Autodesk Inventor part; units mm, degrees
(part 2 of 2)
sketch "Sketch6" plane through (-19, 24.5, 7) normal (0, 0, 1) x (1, 0, 0)
  line L0 (58.5, 3.5) -> (-18, 3.5) projected
  line L1 (-18, 11.1) -> (-18, 3.5) projected
  line L2 (-24, 11.1) -> (-18, 11.1) projected
  line L3 (-24, 11.1) -> (-24, -60.3239) projected
  line L4 (-24, -60.3239) -> (-18, -60.3239) projected
  line L5 (-18, -52.5) -> (-18, -60.3239) projected
  line L6 (-18, -52.5) -> (58.5, -52.5) projected
  arc A0 (58.5, -52.5) -> (61.5, -49.5) centre (58.5, -49.5) ccw projected
  line L7 (61.5, -49.5) -> (61.5, 0.5) projected
  arc A1 (61.5, 0.5) -> (58.5, 3.5) centre (58.5, 0.5) ccw projected
  line L8 (-13.9349, -14.3893) -> (-16.5478, -12.8807) projected
  line L9 (-16.5478, -12.8807) -> (-16.5478, -9.8635) projected
  line L10 (-16.5478, -9.8635) -> (-13.9349, -8.3549) projected
  line L11 (-13.9349, -8.3549) -> (-11.3219, -9.8635) projected
  line L12 (-11.3219, -9.8635) -> (-11.3219, -12.8807) projected
  line L13 (-11.3219, -12.8807) -> (-13.9349, -14.3893) projected
  line L14 (-16.5478, -17.8635) -> (-13.9349, -16.3549) projected
  line L15 (-13.9349, -16.3549) -> (-11.3219, -17.8635) projected
  line L16 (-11.3219, -17.8635) -> (-11.3219, -20.8807) projected
  line L17 (-11.3219, -20.8807) -> (-13.9349, -22.3893) projected
  line L18 (-13.9349, -22.3893) -> (-16.5478, -20.8807) projected
  line L19 (-16.5478, -20.8807) -> (-16.5478, -17.8635) projected
  line L20 (-16.5478, -25.8635) -> (-13.9349, -24.3549) projected
  line L21 (-13.9349, -24.3549) -> (-11.3219, -25.8635) projected
  line L22 (-11.3219, -25.8635) -> (-11.3219, -28.8807) projected
  line L23 (-11.3219, -28.8807) -> (-13.9349, -30.3893) projected
  line L24 (-13.9349, -30.3893) -> (-16.5478, -28.8807) projected
  line L25 (-16.5478, -28.8807) -> (-16.5478, -25.8635) projected
  line L26 (-16.5478, -33.8635) -> (-13.9349, -32.3549) projected
  line L27 (-13.9349, -32.3549) -> (-11.3219, -33.8635) projected
  line L28 (-11.3219, -33.8635) -> (-11.3219, -36.8807) projected
  line L29 (-11.3219, -36.8807) -> (-13.9349, -38.3893) projected
  line L30 (-13.9349, -38.3893) -> (-16.5478, -36.8807) projected
  line L31 (-16.5478, -36.8807) -> (-16.5478, -33.8635) projected
  line L32 (-16.5478, -41.8635) -> (-13.9349, -40.3549) projected
  line L33 (-13.9349, -40.3549) -> (-11.3219, -41.8635) projected
  line L34 (-11.3219, -41.8635) -> (-11.3219, -44.8807) projected
  line L35 (-11.3219, -44.8807) -> (-13.9349, -46.3893) projected
  line L36 (-13.9349, -46.3893) -> (-15.4751, -45.5) projected
  line L37 (-15.4751, -45.5) -> (-16.5, -45.5) projected
  line L38 (-16.5, -45.5) -> (-16.5, -44.9083) projected
  line L39 (-16.5, -44.9083) -> (-16.5478, -44.8807) projected
  line L40 (-16.5478, -44.8807) -> (-16.5478, -41.8635) projected
  line L41 (-8.8465, -45.5) -> (-6.8631, -44.3549) projected
  line L42 (-6.8631, -44.3549) -> (-4.8796, -45.5) projected
  line L43 (-4.8796, -45.5) -> (-8.8465, -45.5) projected
  line L44 (0.0651, -46.3893) -> (-2.5478, -44.8807) projected
  line L45 (-2.5478, -44.8807) -> (-2.5478, -41.8635) projected
  line L46 (-2.5478, -41.8635) -> (0.0651, -40.3549) projected
  line L47 (0.0651, -40.3549) -> (2.6781, -41.8635) projected
  line L48 (2.6781, -41.8635) -> (2.6781, -44.8807) projected
  line L49 (2.6781, -44.8807) -> (0.0651, -46.3893) projected
  line L50 (5.1535, -45.5) -> (7.1369, -44.3549) projected
  line L51 (7.1369, -44.3549) -> (9.1204, -45.5) projected
  line L52 (9.1204, -45.5) -> (5.1535, -45.5) projected
  line L53 (14.0651, -46.3893) -> (11.4522, -44.8807) projected
  line L54 (11.4522, -44.8807) -> (11.4522, -41.8635) projected
  line L55 (11.4522, -41.8635) -> (14.0651, -40.3549) projected
  line L56 (14.0651, -40.3549) -> (16.6781, -41.8635) projected
  line L57 (16.6781, -41.8635) -> (16.6781, -44.8807) projected
  line L58 (16.6781, -44.8807) -> (14.0651, -46.3893) projected
  line L59 (19.1535, -45.5) -> (21.1369, -44.3549) projected
  line L60 (21.1369, -44.3549) -> (23.1204, -45.5) projected
  line L61 (23.1204, -45.5) -> (19.1535, -45.5) projected
  line L62 (28.0651, -46.3893) -> (25.4522, -44.8807) projected
  line L63 (25.4522, -44.8807) -> (25.4522, -41.8635) projected
  line L64 (25.4522, -41.8635) -> (28.0651, -40.3549) projected
  line L65 (28.0651, -40.3549) -> (30.6781, -41.8635) projected
  line L66 (30.6781, -41.8635) -> (30.6781, -44.8807) projected
  line L67 (30.6781, -44.8807) -> (28.0651, -46.3893) projected
  line L68 (33.1535, -45.5) -> (35.1369, -44.3549) projected
  line L69 (35.1369, -44.3549) -> (37.1204, -45.5) projected
  line L70 (37.1204, -45.5) -> (33.1535, -45.5) projected
  line L71 (42.0651, -46.3893) -> (39.4522, -44.8807) projected
  line L72 (39.4522, -44.8807) -> (39.4522, -41.8635) projected
  line L73 (39.4522, -41.8635) -> (42.0651, -40.3549) projected
  line L74 (42.0651, -40.3549) -> (44.6781, -41.8635) projected
  line L75 (44.6781, -41.8635) -> (44.6781, -44.8807) projected
  line L76 (44.6781, -44.8807) -> (42.0651, -46.3893) projected
  line L77 (47.1535, -45.5) -> (49.1369, -44.3549) projected
  line L78 (49.1369, -44.3549) -> (51.1204, -45.5) projected
  line L79 (51.1204, -45.5) -> (47.1535, -45.5) projected
  line L80 (54.5, -45.4856) -> (53.4522, -44.8807) projected
  line L81 (53.4522, -44.8807) -> (53.4522, -41.8635) projected
  line L82 (53.4522, -41.8635) -> (54.5, -41.2585) projected
  line L83 (54.5, -41.2585) -> (54.5, -45.4856) projected
  line L84 (54.5, -37.4856) -> (53.4522, -36.8807) projected
  line L85 (53.4522, -36.8807) -> (53.4522, -33.8635) projected
  line L86 (53.4522, -33.8635) -> (54.5, -33.2585) projected
  line L87 (54.5, -33.2585) -> (54.5, -37.4856) projected
  line L88 (54.5, -29.4856) -> (53.4522, -28.8807) projected
  line L89 (53.4522, -28.8807) -> (53.4522, -25.8635) projected
  line L90 (53.4522, -25.8635) -> (54.5, -25.2585) projected
  line L91 (54.5, -25.2585) -> (54.5, -29.4856) projected
  line L92 (54.5, -21.4856) -> (53.4522, -20.8807) projected
  line L93 (53.4522, -20.8807) -> (53.4522, -17.8635) projected
  line L94 (53.4522, -17.8635) -> (54.5, -17.2585) projected
  line L95 (54.5, -17.2585) -> (54.5, -21.4856) projected
  line L96 (54.5, -13.4856) -> (53.4522, -12.8807) projected
  line L97 (53.4522, -12.8807) -> (53.4522, -9.8635) projected
  line L98 (53.4522, -9.8635) -> (54.5, -9.2585) projected
  line L99 (54.5, -9.2585) -> (54.5, -13.4856) projected
  line L100 (54.5, -5.4856) -> (53.4522, -4.8807) projected
  line L101 (53.4522, -4.8807) -> (53.4522, -3.5) projected
  line L102 (53.4522, -3.5) -> (54.5, -3.5) projected
  line L103 (54.5, -3.5) -> (54.5, -5.4856) projected
  line L104 (44.6781, -3.5) -> (44.6781, -4.8807) projected
  line L105 (44.6781, -4.8807) -> (42.0651, -6.3893) projected
  line L106 (42.0651, -6.3893) -> (39.4522, -4.8807) projected
  line L107 (39.4522, -4.8807) -> (39.4522, -3.5) projected
  line L108 (39.4522, -3.5) -> (44.6781, -3.5) projected
  line L109 (30.6781, -3.5) -> (30.6781, -4.8807) projected
  line L110 (30.6781, -4.8807) -> (28.0651, -6.3893) projected
  line L111 (28.0651, -6.3893) -> (25.4522, -4.8807) projected
  line L112 (25.4522, -4.8807) -> (25.4522, -3.5) projected
  line L113 (25.4522, -3.5) -> (30.6781, -3.5) projected
  line L114 (16.6781, -3.5) -> (16.6781, -4.8807) projected
  line L115 (16.6781, -4.8807) -> (14.0651, -6.3893) projected
  line L116 (14.0651, -6.3893) -> (11.4522, -4.8807) projected
  line L117 (11.4522, -4.8807) -> (11.4522, -3.5) projected
  line L118 (11.4522, -3.5) -> (16.6781, -3.5) projected
  line L119 (2.6781, -3.5) -> (2.6781, -4.8807) projected
  line L120 (2.6781, -4.8807) -> (0.0651, -6.3893) projected
  line L121 (0.0651, -6.3893) -> (-2.5478, -4.8807) projected
  line L122 (-2.5478, -4.8807) -> (-2.5478, -3.5) projected
  line L123 (-2.5478, -3.5) -> (2.6781, -3.5) projected
  line L124 (7.1369, -10.3893) -> (4.524, -8.8807) projected
  line L125 (4.524, -8.8807) -> (4.524, -5.8635) projected
  line L126 (4.524, -5.8635) -> (7.1369, -4.3549) projected
  line L127 (7.1369, -4.3549) -> (9.7499, -5.8635) projected
  line L128 (9.7499, -5.8635) -> (9.7499, -8.8807) projected
  line L129 (9.7499, -8.8807) -> (7.1369, -10.3893) projected
  line L130 (7.1369, -18.3893) -> (4.524, -16.8807) projected
  line L131 (4.524, -16.8807) -> (4.524, -13.8635) projected
  line L132 (4.524, -13.8635) -> (7.1369, -12.3549) projected
  line L133 (7.1369, -12.3549) -> (9.7499, -13.8635) projected
  line L134 (9.7499, -13.8635) -> (9.7499, -16.8807) projected
  line L135 (9.7499, -16.8807) -> (7.1369, -18.3893) projected
  line L136 (-6.8631, -18.3893) -> (-9.476, -16.8807) projected
  line L137 (-9.476, -16.8807) -> (-9.476, -13.8635) projected
  line L138 (-9.476, -13.8635) -> (-6.8631, -12.3549) projected
  line L139 (-6.8631, -12.3549) -> (-4.2501, -13.8635) projected
  line L140 (-4.2501, -13.8635) -> (-4.2501, -16.8807) projected
  line L141 (-4.2501, -16.8807) -> (-6.8631, -18.3893) projected
  line L142 (-6.8631, -10.3893) -> (-9.476, -8.8807) projected
  line L143 (-9.476, -8.8807) -> (-9.476, -5.8635) projected
  line L144 (-9.476, -5.8635) -> (-6.8631, -4.3549) projected
  line L145 (-6.8631, -4.3549) -> (-4.2501, -5.8635) projected
  line L146 (-4.2501, -5.8635) -> (-4.2501, -8.8807) projected
  line L147 (-4.2501, -8.8807) -> (-6.8631, -10.3893) projected
  line L148 (9.7499, -24.8807) -> (7.1369, -26.3893) projected
  line L149 (7.1369, -26.3893) -> (4.524, -24.8807) projected
  line L150 (4.524, -24.8807) -> (4.524, -21.8635) projected
  line L151 (4.524, -21.8635) -> (7.1369, -20.3549) projected
  line L152 (7.1369, -20.3549) -> (9.7499, -21.8635) projected
  line L153 (9.7499, -21.8635) -> (9.7499, -24.8807) projected
  line L154 (9.7499, -32.8807) -> (7.1369, -34.3893) projected
  line L155 (7.1369, -34.3893) -> (4.524, -32.8807) projected
  line L156 (4.524, -32.8807) -> (4.524, -29.8635) projected
  line L157 (4.524, -29.8635) -> (7.1369, -28.3549) projected
  line L158 (7.1369, -28.3549) -> (9.7499, -29.8635) projected
  line L159 (9.7499, -29.8635) -> (9.7499, -32.8807) projected
  line L160 (9.7499, -40.8807) -> (7.1369, -42.3893) projected
  line L161 (7.1369, -42.3893) -> (4.524, -40.8807) projected
  line L162 (4.524, -40.8807) -> (4.524, -37.8635) projected
  line L163 (4.524, -37.8635) -> (7.1369, -36.3549) projected
  line L164 (7.1369, -36.3549) -> (9.7499, -37.8635) projected
  line L165 (9.7499, -37.8635) -> (9.7499, -40.8807) projected
  line L166 (16.6781, -12.8807) -> (14.0651, -14.3893) projected
  line L167 (14.0651, -14.3893) -> (11.4522, -12.8807) projected
  line L168 (11.4522, -12.8807) -> (11.4522, -9.8635) projected
  line L169 (11.4522, -9.8635) -> (14.0651, -8.3549) projected
  line L170 (14.0651, -8.3549) -> (16.6781, -9.8635) projected
  line L171 (16.6781, -9.8635) -> (16.6781, -12.8807) projected
  line L172 (16.6781, -20.8807) -> (14.0651, -22.3893) projected
  line L173 (14.0651, -22.3893) -> (11.4522, -20.8807) projected
  line L174 (11.4522, -20.8807) -> (11.4522, -17.8635) projected
  line L175 (11.4522, -17.8635) -> (14.0651, -16.3549) projected
  line L176 (14.0651, -16.3549) -> (16.6781, -17.8635) projected
  line L177 (16.6781, -17.8635) -> (16.6781, -20.8807) projected
  line L178 (16.6781, -28.8807) -> (14.0651, -30.3893) projected
  line L179 (14.0651, -30.3893) -> (11.4522, -28.8807) projected
  line L180 (11.4522, -28.8807) -> (11.4522, -25.8635) projected
  line L181 (11.4522, -25.8635) -> (14.0651, -24.3549) projected
  line L182 (14.0651, -24.3549) -> (16.6781, -25.8635) projected
  line L183 (16.6781, -25.8635) -> (16.6781, -28.8807) projected
  line L184 (16.6781, -36.8807) -> (14.0651, -38.3893) projected
  line L185 (14.0651, -38.3893) -> (11.4522, -36.8807) projected
  line L186 (11.4522, -36.8807) -> (11.4522, -33.8635) projected
  line L187 (11.4522, -33.8635) -> (14.0651, -32.3549) projected
  line L188 (14.0651, -32.3549) -> (16.6781, -33.8635) projected
  line L189 (16.6781, -33.8635) -> (16.6781, -36.8807) projected
  line L190 (23.7499, -5.8635) -> (23.7499, -8.8807) projected
  line L191 (23.7499, -8.8807) -> (21.1369, -10.3893) projected
  line L192 (21.1369, -10.3893) -> (18.524, -8.8807) projected
  line L193 (18.524, -8.8807) -> (18.524, -5.8635) projected
  line L194 (18.524, -5.8635) -> (21.1369, -4.3549) projected
  line L195 (21.1369, -4.3549) -> (23.7499, -5.8635) projected
  line L196 (18.524, -40.8807) -> (18.524, -37.8635) projected
  line L197 (18.524, -37.8635) -> (21.1369, -36.3549) projected
  line L198 (21.1369, -36.3549) -> (23.7499, -37.8635) projected
  line L199 (23.7499, -37.8635) -> (23.7499, -40.8807) projected
  line L200 (23.7499, -40.8807) -> (21.1369, -42.3893) projected
  line L201 (21.1369, -42.3893) -> (18.524, -40.8807) projected
  line L202 (25.4522, -20.8807) -> (25.4522, -17.8635) projected
  line L203 (25.4522, -17.8635) -> (28.0651, -16.3549) projected
  line L204 (28.0651, -16.3549) -> (30.6781, -17.8635) projected
  line L205 (30.6781, -17.8635) -> (30.6781, -20.8807) projected
  line L206 (30.6781, -20.8807) -> (28.0651, -22.3893) projected
  line L207 (28.0651, -22.3893) -> (25.4522, -20.8807) projected
  line L208 (28.0651, -14.3893) -> (25.4522, -12.8807) projected
  line L209 (25.4522, -12.8807) -> (25.4522, -9.8635) projected
  line L210 (25.4522, -9.8635) -> (28.0651, -8.3549) projected
  line L211 (28.0651, -8.3549) -> (30.6781, -9.8635) projected
  line L212 (30.6781, -9.8635) -> (30.6781, -12.8807) projected
  line L213 (30.6781, -12.8807) -> (28.0651, -14.3893) projected
  line L214 (25.4522, -25.8635) -> (28.0651, -24.3549) projected
  line L215 (28.0651, -24.3549) -> (30.6781, -25.8635) projected
  line L216 (30.6781, -25.8635) -> (30.6781, -28.8807) projected
  line L217 (30.6781, -28.8807) -> (28.0651, -30.3893) projected
  line L218 (28.0651, -30.3893) -> (25.4522, -28.8807) projected
  line L219 (25.4522, -28.8807) -> (25.4522, -25.8635) projected
  line L220 (28.0651, -32.3549) -> (30.6781, -33.8635) projected
  line L221 (30.6781, -33.8635) -> (30.6781, -36.8807) projected
  line L222 (30.6781, -36.8807) -> (28.0651, -38.3893) projected
  line L223 (28.0651, -38.3893) -> (25.4522, -36.8807) projected
  line L224 (25.4522, -36.8807) -> (25.4522, -33.8635) projected
  line L225 (25.4522, -33.8635) -> (28.0651, -32.3549) projected
  line L226 (23.7499, -24.8807) -> (21.1369, -26.3893) projected
  line L227 (21.1369, -26.3893) -> (18.524, -24.8807) projected
  line L228 (18.524, -24.8807) -> (18.524, -21.8635) projected
  line L229 (18.524, -21.8635) -> (21.1369, -20.3549) projected
  line L230 (21.1369, -20.3549) -> (23.7499, -21.8635) projected
  line L231 (23.7499, -21.8635) -> (23.7499, -24.8807) projected
  line L232 (23.7499, -32.8807) -> (21.1369, -34.3893) projected
  line L233 (21.1369, -34.3893) -> (18.524, -32.8807) projected
  line L234 (18.524, -32.8807) -> (18.524, -29.8635) projected
  line L235 (18.524, -29.8635) -> (21.1369, -28.3549) projected
  line L236 (21.1369, -28.3549) -> (23.7499, -29.8635) projected
  line L237 (23.7499, -29.8635) -> (23.7499, -32.8807) projected
  line L238 (23.7499, -16.8807) -> (21.1369, -18.3893) projected
  line L239 (21.1369, -18.3893) -> (18.524, -16.8807) projected
  line L240 (18.524, -16.8807) -> (18.524, -13.8635) projected
  line L241 (18.524, -13.8635) -> (21.1369, -12.3549) projected
  line L242 (21.1369, -12.3549) -> (23.7499, -13.8635) projected
  line L243 (23.7499, -13.8635) -> (23.7499, -16.8807) projected
  line L244 (37.7499, -5.8635) -> (37.7499, -8.8807) projected
  line L245 (37.7499, -8.8807) -> (35.1369, -10.3893) projected
  line L246 (35.1369, -10.3893) -> (32.524, -8.8807) projected
  line L247 (32.524, -8.8807) -> (32.524, -5.8635) projected
  line L248 (32.524, -5.8635) -> (35.1369, -4.3549) projected
  line L249 (35.1369, -4.3549) -> (37.7499, -5.8635) projected
  line L250 (32.524, -40.8807) -> (32.524, -37.8635) projected
  line L251 (32.524, -37.8635) -> (35.1369, -36.3549) projected
  line L252 (35.1369, -36.3549) -> (37.7499, -37.8635) projected
  line L253 (37.7499, -37.8635) -> (37.7499, -40.8807) projected
  line L254 (37.7499, -40.8807) -> (35.1369, -42.3893) projected
  line L255 (35.1369, -42.3893) -> (32.524, -40.8807) projected
  line L256 (39.4522, -20.8807) -> (39.4522, -17.8635) projected
  line L257 (39.4522, -17.8635) -> (42.0651, -16.3549) projected
  line L258 (42.0651, -16.3549) -> (44.6781, -17.8635) projected
  line L259 (44.6781, -17.8635) -> (44.6781, -20.8807) projected
  line L260 (44.6781, -20.8807) -> (42.0651, -22.3893) projected
  line L261 (42.0651, -22.3893) -> (39.4522, -20.8807) projected
  line L262 (42.0651, -14.3893) -> (39.4522, -12.8807) projected
  line L263 (39.4522, -12.8807) -> (39.4522, -9.8635) projected
  line L264 (39.4522, -9.8635) -> (42.0651, -8.3549) projected
  line L265 (42.0651, -8.3549) -> (44.6781, -9.8635) projected
  line L266 (44.6781, -9.8635) -> (44.6781, -12.8807) projected
  line L267 (44.6781, -12.8807) -> (42.0651, -14.3893) projected
  line L268 (39.4522, -25.8635) -> (42.0651, -24.3549) projected
  line L269 (42.0651, -24.3549) -> (44.6781, -25.8635) projected
  line L270 (44.6781, -25.8635) -> (44.6781, -28.8807) projected
  line L271 (44.6781, -28.8807) -> (42.0651, -30.3893) projected
  line L272 (42.0651, -30.3893) -> (39.4522, -28.8807) projected
  line L273 (39.4522, -28.8807) -> (39.4522, -25.8635) projected
  line L274 (42.0651, -32.3549) -> (44.6781, -33.8635) projected
  line L275 (44.6781, -33.8635) -> (44.6781, -36.8807) projected
  line L276 (44.6781, -36.8807) -> (42.0651, -38.3893) projected
  line L277 (42.0651, -38.3893) -> (39.4522, -36.8807) projected
  line L278 (39.4522, -36.8807) -> (39.4522, -33.8635) projected
  line L279 (39.4522, -33.8635) -> (42.0651, -32.3549) projected
  line L280 (37.7499, -24.8807) -> (35.1369, -26.3893) projected
  line L281 (35.1369, -26.3893) -> (32.524, -24.8807) projected
  line L282 (32.524, -24.8807) -> (32.524, -21.8635) projected
  line L283 (32.524, -21.8635) -> (35.1369, -20.3549) projected
  line L284 (35.1369, -20.3549) -> (37.7499, -21.8635) projected
  line L285 (37.7499, -21.8635) -> (37.7499, -24.8807) projected
  line L286 (37.7499, -32.8807) -> (35.1369, -34.3893) projected
  line L287 (35.1369, -34.3893) -> (32.524, -32.8807) projected
  line L288 (32.524, -32.8807) -> (32.524, -29.8635) projected
  line L289 (32.524, -29.8635) -> (35.1369, -28.3549) projected
  line L290 (35.1369, -28.3549) -> (37.7499, -29.8635) projected
  line L291 (37.7499, -29.8635) -> (37.7499, -32.8807) projected
  line L292 (37.7499, -16.8807) -> (35.1369, -18.3893) projected
  line L293 (35.1369, -18.3893) -> (32.524, -16.8807) projected
  line L294 (32.524, -16.8807) -> (32.524, -13.8635) projected
  line L295 (32.524, -13.8635) -> (35.1369, -12.3549) projected
  line L296 (35.1369, -12.3549) -> (37.7499, -13.8635) projected
  line L297 (37.7499, -13.8635) -> (37.7499, -16.8807) projected
  line L298 (51.7499, -5.8635) -> (51.7499, -8.8807) projected
  line L299 (51.7499, -8.8807) -> (49.1369, -10.3893) projected
  line L300 (49.1369, -10.3893) -> (46.524, -8.8807) projected
  line L301 (46.524, -8.8807) -> (46.524, -5.8635) projected
  line L302 (46.524, -5.8635) -> (49.1369, -4.3549) projected
  line L303 (49.1369, -4.3549) -> (51.7499, -5.8635) projected
  line L304 (46.524, -40.8807) -> (46.524, -37.8635) projected
  line L305 (46.524, -37.8635) -> (49.1369, -36.3549) projected
  line L306 (49.1369, -36.3549) -> (51.7499, -37.8635) projected
  line L307 (51.7499, -37.8635) -> (51.7499, -40.8807) projected
  line L308 (51.7499, -40.8807) -> (49.1369, -42.3893) projected
  line L309 (49.1369, -42.3893) -> (46.524, -40.8807) projected
  line L310 (51.7499, -24.8807) -> (49.1369, -26.3893) projected
  line L311 (49.1369, -26.3893) -> (46.524, -24.8807) projected
  line L312 (46.524, -24.8807) -> (46.524, -21.8635) projected
  line L313 (46.524, -21.8635) -> (49.1369, -20.3549) projected
  line L314 (49.1369, -20.3549) -> (51.7499, -21.8635) projected
  line L315 (51.7499, -21.8635) -> (51.7499, -24.8807) projected
  line L316 (51.7499, -32.8807) -> (49.1369, -34.3893) projected
  line L317 (49.1369, -34.3893) -> (46.524, -32.8807) projected
  line L318 (46.524, -32.8807) -> (46.524, -29.8635) projected
  line L319 (46.524, -29.8635) -> (49.1369, -28.3549) projected
  line L320 (49.1369, -28.3549) -> (51.7499, -29.8635) projected
  line L321 (51.7499, -29.8635) -> (51.7499, -32.8807) projected
  line L322 (51.7499, -16.8807) -> (49.1369, -18.3893) projected
  line L323 (49.1369, -18.3893) -> (46.524, -16.8807) projected
  line L324 (46.524, -16.8807) -> (46.524, -13.8635) projected
  line L325 (46.524, -13.8635) -> (49.1369, -12.3549) projected
  line L326 (49.1369, -12.3549) -> (51.7499, -13.8635) projected
  line L327 (51.7499, -13.8635) -> (51.7499, -16.8807) projected
  line L328 (2.6781, -9.8635) -> (2.6781, -12.8807) projected
  line L329 (2.6781, -12.8807) -> (0.0651, -14.3893) projected
  line L330 (0.0651, -14.3893) -> (-2.5478, -12.8807) projected
  line L331 (-2.5478, -12.8807) -> (-2.5478, -9.8635) projected
  line L332 (-2.5478, -9.8635) -> (0.0651, -8.3549) projected
  line L333 (0.0651, -8.3549) -> (2.6781, -9.8635) projected
  line L334 (0.0651, -16.3549) -> (2.6781, -17.8635) projected
  line L335 (2.6781, -17.8635) -> (2.6781, -20.8807) projected
  line L336 (2.6781, -20.8807) -> (0.0651, -22.3893) projected
  line L337 (0.0651, -22.3893) -> (-2.5478, -20.8807) projected
  line L338 (-2.5478, -20.8807) -> (-2.5478, -17.8635) projected
  line L339 (-2.5478, -17.8635) -> (0.0651, -16.3549) projected
  line L340 (-4.2501, -24.8807) -> (-6.8631, -26.3893) projected
  line L341 (-6.8631, -26.3893) -> (-9.476, -24.8807) projected
  line L342 (-9.476, -24.8807) -> (-9.476, -21.8635) projected
  line L343 (-9.476, -21.8635) -> (-6.8631, -20.3549) projected
  line L344 (-6.8631, -20.3549) -> (-4.2501, -21.8635) projected
  line L345 (-4.2501, -21.8635) -> (-4.2501, -24.8807) projected
  line L346 (2.6781, -25.8635) -> (2.6781, -28.8807) projected
  line L347 (2.6781, -28.8807) -> (0.0651, -30.3893) projected
  line L348 (0.0651, -30.3893) -> (-2.5478, -28.8807) projected
  line L349 (-2.5478, -28.8807) -> (-2.5478, -25.8635) projected
  line L350 (-2.5478, -25.8635) -> (0.0651, -24.3549) projected
  line L351 (0.0651, -24.3549) -> (2.6781, -25.8635) projected
  line L352 (2.6781, -33.8635) -> (2.6781, -36.8807) projected
  line L353 (2.6781, -36.8807) -> (0.0651, -38.3893) projected
  line L354 (0.0651, -38.3893) -> (-2.5478, -36.8807) projected
  line L355 (-2.5478, -36.8807) -> (-2.5478, -33.8635) projected
  line L356 (-2.5478, -33.8635) -> (0.0651, -32.3549) projected
  line L357 (0.0651, -32.3549) -> (2.6781, -33.8635) projected
  line L358 (-4.2501, -29.8635) -> (-4.2501, -32.8807) projected
  line L359 (-4.2501, -32.8807) -> (-6.8631, -34.3893) projected
  line L360 (-6.8631, -34.3893) -> (-9.476, -32.8807) projected
  line L361 (-9.476, -32.8807) -> (-9.476, -29.8635) projected
  line L362 (-9.476, -29.8635) -> (-6.8631, -28.3549) projected
  line L363 (-6.8631, -28.3549) -> (-4.2501, -29.8635) projected
  line L364 (-4.2501, -37.8635) -> (-4.2501, -40.8807) projected
  line L365 (-4.2501, -40.8807) -> (-6.8631, -42.3893) projected
  line L366 (-6.8631, -42.3893) -> (-9.476, -40.8807) projected
  line L367 (-9.476, -40.8807) -> (-9.476, -37.8635) projected
  line L368 (-9.476, -37.8635) -> (-6.8631, -36.3549) projected
  line L369 (-6.8631, -36.3549) -> (-4.2501, -37.8635) projected
  line L370 (-11.3219, -3.5) -> (-11.3219, -4.8807) projected
  line L371 (-11.3219, -4.8807) -> (-13.9349, -6.3893) projected
  line L372 (-13.9349, -6.3893) -> (-16.5, -4.9083) projected
  line L373 (-16.5, -4.9083) -> (-16.5, -3.5) projected
  line L374 (-16.5, -3.5) -> (-11.3219, -3.5) projected
  line L375 (-18, 11.1) -> (3.1939, 3.5)
  line L376 (-18, 3.5) -> (-18, -52.5) construction
  line L377 (-18, -24.5) -> (-16.3532, -24.5) construction
  line L378 (3.1939, 3.5) -> (3.1939, -52.5) construction
  line L379 (3.1939, -52.5) -> (-18, -60.3239)
  point P0 (19, -24.5)
  constraints: 10 end point, 2 point on line, 1 horizontal, 1 midpoint, 1 perpendicular, 1 vertical
extrude "Extrusion5" add sketch "Sketch6" against normal up to surface (3 mm away) contours L0 L1 L375 | L379 L5 L6
chamfer "Chamfer1" distance 1 angle 45 10 edges at (-26.4031, 31.8, 7) (11.8469, 28, 7) (41.6213, 27.1213, 7) (42.5, 0, 7) (41.6213, -27.1213, 7) (11.8469, -28, 7) (-26.4031, -31.912, 7) (-40, -35.8239, 7) (-40, 35.6, 7) (-43, -0.112, 7)
fillet "Fillet1" radius 3.175 2 edges at (-40, -28, 4) (-40, 28, 4)
body "Solid1"
